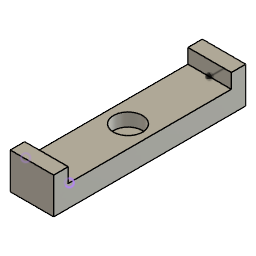
gearbox_side_mount (Autodesk Fusion 360 design; units mm, degrees)
Autodesk Fusion 360 part; units mm, degrees
sketch "Sketch1" plane through (0, 0, 0) normal (0, 1, 0) x (1, 0, 0)
  line L0 (0, 0) -> (-6.6, 0)
  line L1 (-6.6, 0) -> (-6.6, -26.6)
  line L2 (-6.6, -26.6) -> (0, -26.6)
  line L3 (0, -26.6) -> (0, 0)
  dimension "d1" = 6.6
  dimension "d2" = 26.6
  constraint horizontal L0
  constraint vertical L1
  constraint horizontal L2
  constraint vertical L3
  constraint coincident L0.start L3.end
  measures "d1" distance of L0.start L0.end
  measures "d2" distance of L0.start L2.end
sketch "Sketch2" plane through (0, 3.4, 0) normal (0, 1, 0) x (-1, 0, 0)
  line L0 (0, 26.6) -> (0, 0)
  line L1 (0, 0) -> (6.6, 0)
  line L2 (6.6, 0) -> (6.6, 26.6)
  line L3 (6.6, 26.6) -> (0, 26.6)
  circle A0 centre (3.3, 13.3) radius 2
  dimension "d5" = 4
  measures "d5" diameter of A0
sketch "Sketch3" plane through (0, 0, 0) normal (0, 1, 0) x (1, 0, 0)
  line L0 (0, 0) -> (-6, 0)
  line L1 (-6, 0) -> (-6, -26.5)
  line L2 (-6, -26.5) -> (0, -26.5)
  line L3 (0, -26.5) -> (0, 0)
  dimension "d9" = 6
  dimension "d10" = 26.5
  constraint horizontal L0
  constraint vertical L1
  constraint horizontal L2
  constraint vertical L3
  constraint coincident L0.start L3.end
  measures "d9" distance of L0.start L0.end
  measures "d10" distance of L0.start L2.end
extrude "Extrude2" add sketch "Sketch3" along normal blind 3
sketch "Sketch4" plane through (0, 3, 0) normal (0, 1, 0) x (-1, 0, 0)
  line L0 (0, 26.5) -> (0, 0)
  line L1 (0, 0) -> (6, 0)
  line L2 (6, 0) -> (6, 26.5)
  line L3 (6, 26.5) -> (0, 26.5)
  line L4 (3, 24.35) -> (6, 24.35)
  line L5 (3, 24.35) -> (0, 24.35)
  constraint coincident L2 L4.end
  constraint perpendicular L2 L4
  constraint coincident L0 L5.end
  constraint perpendicular L0 L5
extrude "Extrude3" add sketch "Sketch4" along normal blind 5 contours L0 L2 L3 L4 L5
sketch "Sketch5" plane through (0, 3, 0) normal (0, 1, 0) x (-1, 0, 0)
  line L0 (0, 24.35) -> (0, 0)
  line L1 (0, 0) -> (6, 0)
  line L2 (6, 0) -> (6, 24.35)
  line L3 (3, 0) -> (3, 2)
  dimension "d16" = 2
  constraint midpoint L1 L3.start
  constraint perpendicular L1 L3
  measures "d16" distance of L3.start L3.end
extrude "Extrude4" cut 1 faces at (-2, 8, 25.7833) along direction (0, -1, 0) blind 5
sketch "Sketch6" plane through (0, 3, 0) normal (0, 1, 0) x (-1, 0, 0)
  line L0 (0, 26.5) -> (0, 0)
  line L1 (0, 0) -> (6, 0)
  line L2 (6, 0) -> (6, 26.5)
  line L3 (6, 26.5) -> (0, 26.5)
  line L4 (6, 2) -> (0, 2)
  line L5 (2.5, 24.5) -> (2.6614, 24.5)
  line L6 (2.6614, 24.5) -> (6, 24.5)
  line L7 (2.5, 24.5) -> (0, 24.5)
  constraint coincident L2 L4.start
  constraint coincident L0 L4.end
  constraint perpendicular L0 L4
  constraint coincident L2 L6.end
  constraint perpendicular L2 L6
  constraint coincident L0 L7.end
  constraint perpendicular L0 L7
extrude "Extrude5" add sketch "Sketch6" along normal blind 5 contours L0 L2 L3 L5 L6 L7 | L0 L1 L2 L4
sketch "Sketch7" plane through (0, 3, 0) normal (0, 1, 0) x (-1, 0, 0)
  line L0 (0, 2) -> (6, 2)
  line L1 (6, 2) -> (6, 24.5)
  line L2 (6, 24.5) -> (0, 24.5)
  line L3 (0, 24.5) -> (0, 2)
  circle A0 centre (3, 13.25) radius 2
  dimension "d22" = 4
  measures "d22" diameter of A0
hole "Hole2" at (-3, 3, 13.25) direction (0, -1, 0) diameter 4 depth 1.6 tip angle 180
move_face "OffsetFaces1" offset -0.1 1 faces at (-3.4967, 1.4, 13.1618)
move_face "OffsetFaces2" offset 0.05 1 faces at (-3.4967, 1.3, 13.1618)
move_face "OffsetFaces3" offset -0.05 1 faces at (-3.4967, 1.35, 13.1618)
move_face "OffsetFaces4" offset -0.1 1 faces at (-3.4967, 1.3, 13.1618)
move_face "OffsetFaces5" offset -3 2 faces at (-4, 8, 25.1667) (-2, 8, 1.3333)
equation "d16 = ( ( 26.5 - 22.5 ) / 2 ) * 1 mm"
equation "d23 = 20.4 mm - 18.8 mm"
